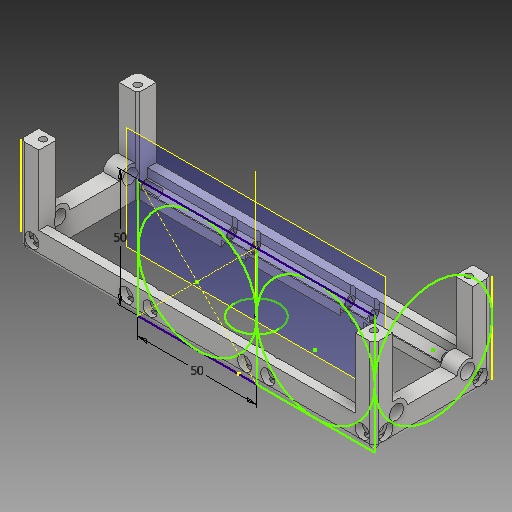
# Autodesk Inventor part: 10_Cube_2x_v0
Saved by Autodesk Inventor 2019 (Build 230136000, 136)
## iProperties
Created: 2018-05-19
Part Number: 10_Cube_2x_v0
Material: Generisch
Document SubType Name: Modeling
Designer: diederichbenedict
Density: 1 g/cm^3
Appearance: Vorgabe
Mass: 20.3218 g
Surface Area: 129.075 cm^2
Volume: 20.3218 cm^3
Author: diederichbenedict
Autodesk Inventor part; units mm, degrees
ref_plane "YZ Plane" through (0, 0, 0) normal (1, 0, 0) x (0, 1, 0)
ref_plane "XZ Plane" through (0, 0, 0) normal (0, 1, 0) x (-1, 0, 0)
sketch "Skizze1" plane through (0, 0, 0) normal (0, 0, 1) x (1, 0, 0)
  line L0 (-74.9, 24.9) -> (74.9, 24.9)
  line L1 (74.9, 24.9) -> (74.9, -24.9)
  line L2 (74.9, -24.9) -> (-74.9, -24.9)
  line L3 (-74.9, -24.9) -> (-74.9, 24.9)
  line L4 (-74.9, 24.9) -> (74.9, -24.9) construction
  line L5 (74.9, 24.9) -> (-74.9, -24.9) construction
  line L6 (66.9528, -17.9) -> (-66.9528, -17.9)
  line L7 (-67.9, -16.9528) -> (-67.9, 16.9528)
  line L8 (-66.9528, 17.9) -> (66.9528, 17.9)
  line L9 (67.9, 16.9528) -> (67.9, -16.9528)
  line L10 (20.5, -20.5) -> (-20.5, 20.5) construction
  line L11 (-20.5, -20.5) -> (20.5, 20.5) construction
  line L12 (-66.9528, 17.9) -> (-67.9, 16.9528)
  line L13 (-66.9528, 17.9) -> (-65.6133, 17.9) construction
  line L14 (67.9, -16.9528) -> (66.9528, -17.9)
  line L15 (67.9, -16.9528) -> (69.2395, -16.9528) construction
  line L16 (-67.9, -16.9528) -> (-66.9528, -17.9)
  line L17 (66.9528, 17.9) -> (67.9, 16.9528)
  point P0 (0, 0)
  dimension "d0" = 149.8
  dimension "d1" = 49.8
  dimension "d2" = 41
  dimension "d3" = 41
  dimension "d4" = 135
  dimension "d5" = 60
  dimension "d6" = 135
  dimension "d7" = 60
  dimension "a1" = 60
  dimension "d9" = 60
  dimension "a2" = 7
  dimension "d42" = 7
  dimension "d43" = 7
  dimension "d44" = 7
  constraints: 36 end point, 4 horizontal, 4 midpoint, 4 parallel, 4 perpendicular, 2 equal length
  measures "d0" distance of L1.end L2.end
  measures "d1" distance of L0.end L1.end
  measures "d2" distance of L10.end L11.end
  measures "d3" distance of L11.start L10.end
  measures "d4" angle of L12 L13
  measures "d5" distance from line of point (0, 0) L12
  measures "d6" angle of L14 L15
  measures "d7" distance from line of point (0, 0) L14
  measures "a1" distance from line of point (0, 0) L17
  measures "d9" distance from line of L16 point (0, 0)
  measures "a2" distance between parallel lines of L8 L0
  measures "d42" distance between parallel lines of L3 L7
  measures "d43" distance between parallel lines of L2 L6
  measures "d44" distance between parallel lines of L1 L9
extrude "Extrusion1" add sketch "Skizze1" along normal blind 10.3
sketch "Skizze2" plane through (0, 0, 10.3) normal (0, 0, 1) x (1, 0, 0)
  line L0 (-67.9, 16.9528) -> (-66.9528, 17.9) construction
  line L1 (-66.9528, 17.9) -> (66.9528, 17.9) construction
  line L2 (66.9528, 17.9) -> (67.9, 16.9528) construction
  line L3 (67.9, 16.9528) -> (67.9, -16.9528) construction
  line L4 (67.9, -16.9528) -> (66.9528, -17.9) construction
  line L5 (66.9528, -17.9) -> (-66.9528, -17.9) construction
  line L6 (-66.9528, -17.9) -> (-67.9, -16.9528) construction
  line L7 (-67.9, -16.9528) -> (-67.9, 16.9528) construction
  line L8 (74.9, 24.9) -> (-74.9, 24.9) construction
  line L9 (-74.9, 24.9) -> (-74.9, -24.9) construction
  line L10 (-74.9, -24.9) -> (74.9, -24.9) construction
  line L11 (74.9, -24.9) -> (74.9, 24.9) construction
  line L12 (-67.9, -16.9528) -> (-74.9, -16.9528)
  line L13 (-74.9, -24.9) -> (-74.9, 24.9) projected
  line L14 (-74.9, -16.9528) -> (-74.9, -24.9)
  line L15 (-67.9, -16.9528) -> (-66.9528, -17.9) projected
  line L16 (-67.9, -16.9528) -> (-66.9528, -17.9)
  line L17 (-66.9528, -17.9) -> (-66.9528, -24.9)
  line L18 (74.9, -24.9) -> (-74.9, -24.9) projected
  line L19 (-74.9, -24.9) -> (-66.9528, -24.9)
  line L20 (-17.9, -14.9) -> (-17.9, 14.9) projected
  line L21 (14.9, -17.9) -> (-14.9, -17.9) projected
  line L22 (17.9, 14.9) -> (17.9, -14.9) projected
  line L23 (-14.9, 17.9) -> (-9.9, 17.9) projected
  circle A0 centre (0, 0) radius 17.9
  line L24 (66.9528, -17.9) -> (67.9, -16.9528)
  line L25 (67.9, -16.9528) -> (74.9, -16.9528)
  line L26 (74.9, -24.9) -> (74.9, -16.9528)
  line L27 (66.9528, -24.9) -> (74.9, -24.9)
  line L28 (66.9528, -17.9) -> (66.9528, -24.9)
  line L29 (67.9, 16.9528) -> (66.9528, 17.9)
  line L30 (66.9528, 17.9) -> (66.9528, 24.9)
  line L31 (74.9, 24.9) -> (66.9528, 24.9)
  line L32 (74.9, 16.9528) -> (74.9, 24.9)
  line L33 (67.9, 16.9528) -> (74.9, 16.9528)
  line L34 (-66.9528, 17.9) -> (-67.9, 16.9528)
  line L35 (-67.9, 16.9528) -> (-74.9, 16.9528)
  line L36 (-74.9, 24.9) -> (-74.9, 16.9528)
  line L37 (-66.9528, 24.9) -> (-74.9, 24.9)
  line L38 (-66.9528, 17.9) -> (-66.9528, 24.9)
  line L39 (0, 0) -> (49.9, -49.9) construction
  line L40 (27.2236, -28.6378) -> (29.3449, -30.7591)
  line L41 (29.3449, -30.7591) -> (30.7591, -29.3449)
  line L42 (30.7591, -29.3449) -> (28.6378, -27.2236)
  line L43 (28.6378, -27.2236) -> (27.2236, -28.6378)
  line L44 (27.2236, -28.6378) -> (30.7591, -29.3449) construction
  line L45 (29.3449, -30.7591) -> (28.6378, -27.2236) construction
  line L46 (66.9528, -17.9) -> (67.9, -16.9528) projected
  point P0 (28.9914, -28.9914)
  point P1 (43.1335, -41.7193)
  point P2 (41.7193, -43.1335)
  dimension "d80" = 360
  dimension "d101" = 3
  dimension "d102" = 2
  constraints: 54 end point, 8 point on line, 3 perpendicular, 3 tangent, 2 collinear, 2 midpoint, 2 parallel, 1 centre point, 1 vertical, 3 other
  measures "d101" distance of L40.start L40.end
  measures "d102" distance of L41.end L40.end
extrude "Extrusion2" add sketch "Skizze2" along normal blind 29.4 contours L15 L17 L18 L13 L12 | L13 L37 L38 L34 L35 | L18 L28 L24 L25 L26 | L29 L30 L31 L32 L33
fillet "Rundung1" radius 2 8 edges at (74.9, 24.9, 19.85) (74.9, 0, 0) (74.9, -24.9, 19.85) (-74.9, 24.9, 19.85) (-74.9, -24.9, 19.85) (-74.9, 0, 0) (0, -24.9, 0) (0, 24.9, 0)
sketch "Skizze3" plane through (0, 0, 39.7) normal (0, 0, 1) x (1, 0, 0)
  line L0 (70, 20) -> (-70, 20) construction
  line L1 (-70, 20) -> (-70, -20) construction
  line L2 (-70, -20) -> (70, -20) construction
  line L3 (70, -20) -> (70, 20) construction
  line L4 (70, 20) -> (-70, -20) construction
  line L5 (-70, 20) -> (70, -20) construction
  line L6 (22.9, -22.9) -> (20.7681, -22.9) projected
  line L7 (22.9, -20.7681) -> (22.9, -22.9) projected
  arc A0 (20.7681, -22.9) -> (22.9, -20.7681) centre (20, -20) ccw projected
  point P0 (0, 0)
  point P1 (-20, 20)
  point P2 (-20, 20)
  point P3 (-20, 20)
  point P4 (20, -20)
  point P5 (20, -20)
  point P6 (-20, -20)
  point P7 (-20, 20)
  point P8 (20, -20)
  point P9 (-20, -20)
  point P10 (-20, 20)
  point P11 (-20, -20)
  point P12 (-20, 20)
  point P13 (-20, -20)
  point P14 (-20, 20)
  point P15 (-15.7881, 5.2)
  point P16 (-15.7881, -5.2)
  dimension "d15" = 140
  dimension "d16" = 40
  constraints: 12 end point, 2 midpoint, 2 parallel, 1 horizontal, 1 perpendicular
  measures "d15" distance of L2.end L1.end
  measures "d16" distance of L1.end L0.end
hole "Bohrung1" at (70, -20, 39.7) at (-70, -20, 39.7) at (-70, 20, 39.7) at (70, 20, 39.7) direction (0, 0, -1) diameter 2.9 depth 10 tip angle 118
sketch "Skizze4" plane through (0, 0, 0) normal (0, 0, -1) x (-1, 0, 0)
  line L0 (66.9528, 17.9) -> (67.9, 16.9528) projected
  line L1 (67.9, 16.9528) -> (67.9, -16.9528) projected
  line L2 (67.9, -16.9528) -> (66.9528, -17.9) projected
  line L3 (66.9528, -17.9) -> (-66.9528, -17.9) projected
  line L4 (-66.9528, -17.9) -> (-67.9, -16.9528) projected
  line L5 (-67.9, -16.9528) -> (-67.9, 16.9528) projected
  line L6 (-67.9, 16.9528) -> (-66.9528, 17.9) projected
  line L7 (-66.9528, 17.9) -> (66.9528, 17.9) projected
  line L8 (-72.9, 22.9) -> (72.9, 22.9) projected
  line L9 (-72.9, -22.9) -> (-72.9, 22.9) projected
  line L10 (72.9, -22.9) -> (-72.9, -22.9) projected
  line L11 (72.9, 22.9) -> (72.9, -22.9) projected
  line L12 (-70, 20) -> (70, 20) construction
  line L13 (70, 20) -> (70, -20) construction
  line L14 (70, -20) -> (-70, -20) construction
  line L15 (-70, -20) -> (-70, 20) construction
  line L16 (-70, 20) -> (70, -20) construction
  line L17 (70, 20) -> (-70, -20) construction
  line L18 (70, 20) -> (30, 20) construction
  line L19 (30, 20) -> (30, -20) construction
  line L20 (30, -20) -> (70, -20) construction
  line L21 (70, -20) -> (70, 20) construction
  line L22 (-70, 20) -> (-30, 20) construction
  line L23 (-30, 20) -> (-30, -20) construction
  line L24 (-30, -20) -> (-70, -20) construction
  line L25 (-70, -20) -> (-70, 20) construction
  line L26 (-30, -20) -> (30, -20) construction
  line L27 (30, -20) -> (30, 20) construction
  line L28 (30, 20) -> (-30, 20) construction
  line L29 (-30, 20) -> (-30, -20) construction
  line L30 (20, 20) -> (-20, 20) construction
  line L31 (-20, 20) -> (-20, -20) construction
  line L32 (-20, -20) -> (20, -20) construction
  line L33 (20, -20) -> (20, 20) construction
  line L34 (20, 20) -> (-20, -20) construction
  line L35 (-20, 20) -> (20, -20) construction
  point P0 (0, 0)
  dimension "d149" = 140
  dimension "d150" = 40
  dimension "d151" = 40
  dimension "d152" = 40
  dimension "d153" = 40
  dimension "d154" = 40
  constraints: 48 end point, 10 parallel, 5 horizontal, 5 perpendicular, 4 midpoint, 2 point on line
  measures "d149" distance of L13.end L14.end
  measures "d150" distance of L12.end L13.end
  measures "d151" distance of L20.end L19.end
  measures "d152" distance of L23.end L24.end
  measures "d153" distance of L32.end L31.end
  measures "d154" distance of L31.end L30.end
hole "Bohrung2" at (-70, 20, 0) at (-70, -20, 0) at (-30, -20, 0) at (-20, -20, 0) at (-30, 20, 0) at (-20, 20, 0) at (20, 20, 0) at (30, 20, 0) at (70, 20, 0) at (70, -20, 0) at (30, -20, 0) at (20, -20, 0) direction (0, 0, 1) diameter 3 depth 15 tip angle 118 counterbore diameter 6.2 counterbore depth 2.5
sketch "Skizze8" plane through (74.9, -16.9528, 10.3) normal (1, 0, 0) x (0, 0, -1)
  line L0 (8.3, 41.8528) -> (-29.4, 41.8528) projected
  line L1 (10.3, 38.0483) -> (10.3, 39.8528) projected
  line L2 (10.3, 39.8528) -> (8.3, 39.8528) projected
  line L3 (8.3, 39.8528) -> (8.3, -5.9472) projected
  line L4 (8.3, -5.9472) -> (10.3, -5.9472) projected
  line L5 (10.3, -5.9472) -> (10.3, -4.1426) projected
  line L6 (10.3, -1.9517) -> (10.3, 35.8574) projected
  line L7 (-29.4, -7.9472) -> (8.3, -7.9472) projected
  circle A0 centre (-14.6, 16.9528) radius 24.9 construction
  line L8 (-34.6, -3.0472) -> (5.4, -3.0472) construction
  line L9 (5.4, -3.0472) -> (5.4, 36.9528) construction
  line L10 (5.4, 36.9528) -> (-34.6, 36.9528) construction
  line L11 (-34.6, 36.9528) -> (-34.6, -3.0472) construction
  line L12 (-34.6, -3.0472) -> (5.4, 36.9528) construction
  line L13 (5.4, -3.0472) -> (-34.6, 36.9528) construction
  point P0 (-34.7, -4.2101)
  point P1 (5.3, 35.7899)
  point P2 (5.3, -4.2101)
  point P3 (-34.7, 35.7899)
  dimension "d155" = 40
  dimension "d156" = 40
  constraints: 12 end point, 3 tangent, 2 midpoint, 2 parallel, 2 vertical alignment, 1 centre point, 1 horizontal, 1 perpendicular
  measures "d155" distance of L10.end L9.end
  measures "d156" distance of L9.end L8.end
sketch "Skizze9" plane through (66.9528, 17.9, 10.3) normal (-1, 0, 0) x (0, 0, 1)
  line L0 (-3.2288, -37.966) -> (32.6288, -37.966) construction
  line L1 (32.6288, -37.966) -> (34.766, -35.8288) construction
  line L2 (34.766, -35.8288) -> (34.766, 0.0288) construction
  line L3 (34.766, 0.0288) -> (32.6288, 2.166) construction
  line L4 (32.6288, 2.166) -> (-3.2288, 2.166) construction
  line L5 (-3.2288, 2.166) -> (-5.366, 0.0288) construction
  line L6 (-5.366, 0.0288) -> (-5.366, -35.8288) construction
  line L7 (-5.366, -35.8288) -> (-3.2288, -37.966) construction
  circle A0 centre (29.7, -2.9) radius 3.2639 construction
  circle A1 centre (-0.3, -2.9) radius 3.2639 construction
  circle A2 centre (-0.3, -32.9) radius 3.2639 construction
  circle A3 centre (29.7, -32.9) radius 3.2639 construction
  circle A4 centre (14.7, -17.9) radius 13.3985 construction
  line L8 (-3.643, 3.166) -> (33.043, 3.166)
  line L9 (33.043, 3.166) -> (35.766, 0.443)
  line L10 (35.766, 0.443) -> (35.766, -36.243)
  line L11 (35.766, -36.243) -> (33.043, -38.966)
  line L12 (33.043, -38.966) -> (-3.643, -38.966)
  line L13 (-3.643, -38.966) -> (-6.366, -36.243)
  line L14 (-6.366, -36.243) -> (-6.366, 0.443)
  line L15 (-6.366, 0.443) -> (-3.643, 3.166)
  point P0 (-10.3, -17.9)
  dimension "d82" = 1
  constraints: 16 end point, 7 other
  measures "d82" distance between parallel lines of L4 L8
extrude "Extrusion5" cut sketch "Skizze9" along normal up to surface (133.9056 mm away)
sketch "Skizze10" plane through (-74.9, -16.9528, 10.3) normal (-1, 0, 0) x (0, 0, 1)
  circle A0 centre (-0.4, 31.4969) radius 3.0099 construction
  circle A1 centre (-0.4, 31.4969) radius 3.0099 projected
  circle A2 centre (-0.4, 1.497) radius 3.0099 projected
extrude "Extrusion6" cut sketch "Skizze10" against normal through all
sketch "Skizze11" plane through (-74.9, -22.9, 2) normal (-1, 0, 0) x (0, 0, 1)
  arc A0 (9.7049, 39.8528) -> (8.3, 34.4609) centre (7.9, 37.4441) ccw construction
  line L0 (9.7049, 39.8528) -> (37.7, 39.8528) construction
  line L1 (37.7, 45.8) -> (37.7, 39.8528) construction
  line L2 (0, 45.8) -> (37.7, 45.8) construction
  line L3 (0, 0) -> (0, 45.8) construction
  line L4 (37.7, 0) -> (0, 0) construction
  line L5 (37.7, 5.9472) -> (37.7, 0) construction
  line L6 (10.5113, 5.9472) -> (37.7, 5.9472) construction
  arc A1 (8.3, 10.4274) -> (10.5113, 5.9472) centre (7.9, 7.4442) ccw construction
  line L7 (8.3, 34.4609) -> (8.3, 10.4274) construction
  arc A2 (8.3, 34.4609) -> (9.7049, 39.8528) centre (7.9, 37.4441) ccw
  line L8 (10.5113, 5.9472) -> (37.7, 5.9472) projected
  line L9 (9.7049, 39.8528) -> (37.7, 39.8528) projected
  arc A3 (8.3, 33.1135) -> (11.5212, 39.8528) centre (7.9, 37.4441) ccw
  line L10 (8.3, 34.4609) -> (8.3, 10.4274) projected
  line L11 (8.3, 33.1135) -> (8.3, 34.4609)
  line L12 (11.5212, 39.8528) -> (9.7049, 39.8528)
  line L13 (8.3, 10.4274) -> (8.3, 34.4609) projected
  arc A4 (10.5113, 5.9472) -> (8.3, 10.4274) centre (7.9, 7.4442) ccw
  arc A5 (12.3275, 5.9472) -> (8.3, 12.1007) centre (7.9, 7.4442) ccw
  line L14 (8.3, 12.1007) -> (8.3, 10.4274)
  line L15 (12.3275, 5.9472) -> (10.5113, 5.9472)
  constraints: 9 point on circle, 8 end point, 4 centre point, 3 coincident, 2 collinear, 2 horizontal, 2 point on line
extrude "Extrusion7" add sketch "Skizze11" against normal up to surface (7 mm away)
sketch "Skizze12" plane through (74.9, -22.9, 2) normal (1, 0, 0) x (0, 0, -1)
  line L0 (-10.5113, 5.9472) -> (-37.7, 5.9472) projected
  arc A0 (-9.7049, 39.8528) -> (-6.0951, 39.8528) centre (-7.9, 37.4441) ccw projected
  line L1 (-9.7049, 39.8528) -> (-11.5212, 39.8528) projected
  arc A1 (-11.5212, 39.8528) -> (-8.3, 33.1135) centre (-7.9, 37.4441) ccw projected
  line L2 (-8.3, 12.1007) -> (-8.3, 33.1135) projected
  arc A2 (-8.3, 12.1007) -> (-12.3275, 5.9472) centre (-7.9, 7.4442) ccw projected
  line L3 (-10.5113, 5.9472) -> (-12.3275, 5.9472) projected
  arc A3 (-5.2888, 5.9472) -> (-10.5113, 5.9472) centre (-7.9, 7.4442) ccw projected
  line L4 (2, 5.9472) -> (-5.2888, 5.9472) projected
  line L5 (2, 39.8528) -> (2, 5.9472) projected
  line L6 (2, 39.8528) -> (-6.0951, 39.8528) projected
  line L7 (-8.3, 10.4274) -> (-8.3, 34.4609) projected
  point P0 (-8.3, -17.1828)
  constraints: 1 other
ref_plane "Arbeitsebene1" through (17.9, -21.066, 43) normal (-1, 0, 0) x (0, 0, 1)
extrude "Extrusion8" add sketch "Skizze12" against normal up to surface (7 mm away) contours L0 A2 L7 A3 | A1 L1 A0 L7
hole "Bohrung3" at (74.9, -21.163, 45) at (74.9, 18.837, 45) at (74.9, -20, 4.9) at (74.9, 20, 4.9) direction (-1, 0, 0) diameter 3 depth 15 tip angle 118 counterbore diameter 6.2 counterbore depth 2.5
sketch "Skizze14" plane through (0, 0, 0) normal (0, 0, -1) x (-1, 0, 0)
  circle A0 centre (0, 0) radius 9.428
  constraints: 1 centre point, 1 coincident
pattern_circular "Runde Anordnung3" count 2 over 360 about axis through (0, 0, 0) along (0, 0, 1) of "Bohrung3"
sketch "Skizze15" plane through (-66.9528, 24.9, 10.3) normal (0, 1, 0) x (1, 0, 0)
  line L0 (87.0528, -63.0868) -> (-2.9472, -63.0868) construction
  line L1 (-2.9472, -63.0868) -> (-2.9472, 5.25) construction
  line L2 (-2.9472, 5.25) -> (87.0528, 5.25) construction
  line L3 (87.0528, 5.25) -> (87.0528, -63.0868) construction
  line L4 (87.0528, -63.0868) -> (-2.9472, 5.25) construction
  line L5 (-2.9472, -63.0868) -> (87.0528, 5.25) construction
  circle A0 centre (-2.9472, 5.25) radius 2.5 construction
  circle A1 centre (87.0528, 5.25) radius 2.5 construction
  circle A2 centre (47.0528, 5.25) radius 2.5 construction
  circle A3 centre (37.0528, 5.25) radius 2.5 construction
  circle A4 centre (96.8528, 5.25) radius 2.9342
  circle A5 centre (136.8528, 5.25) radius 4.1581
  line L6 (141.8528, 8.3) -> (141.8528, 2.3) projected
  line L7 (-7.9472, 4.3046) -> (-7.9472, -29.4) projected
  point P0 (66.9528, 10.3)
  point P1 (42.0528, -28.9184)
  point P2 (141.8528, 4.3046)
  dimension "d134" = 90
  dimension "d135" = 5
  dimension "d136" = 5
  dimension "d137" = 5
  dimension "d138" = 5
  dimension "d139" = 40
  dimension "d140" = 40
  dimension "d157" = 5
  dimension "d158" = 40
  dimension "d159" = 5
  constraints: 12 end point, 6 centre point, 2 coincident, 2 midpoint, 2 parallel, 2 point on line, 1 horizontal, 1 perpendicular
  measures "d134" distance of L1.end L2.end
  measures "d135" diameter of A0
  measures "d136" diameter of A1
  measures "d137" diameter of A2
  measures "d138" diameter of A3
  measures "d139" distance from line of A3.centre L1
  measures "d140" distance from line of A2.centre L3
  measures "d157" distance from line of A5.centre L6
  measures "d158" distance of A4.centre A5.centre
  measures "d159" distance from line of L1.end L7
hole "Bohrung4" at (20.1, 24.9, 5.05) at (-19.9, 24.9, 5.05) at (-29.9, 24.9, 5.05) at (-69.9, 24.9, 5.05) at (29.9, 24.9, 5.05) at (69.9, 24.9, 5.05) direction (0, -1, 0) diameter 3 depth 8 tip angle 118 counterbore diameter 6 counterbore depth 3
ref_plane "Arbeitsebene2" through (0, 0, 0) normal (0, 1, 0) x (1, 0, 0)
mirror "Spiegeln1" about plane through (0, 0, 0) normal (0, 1, 0) of "Bohrung4"
sketch "Skizze16" plane through (74.9, 16.9528, 39.7) normal (1, 0, 0) x (0, 0, -1)
  line L0 (0, -41.8528) -> (37.7, -41.8528) projected
  line L1 (37.7, 7.9472) -> (0, 7.9472) projected
  circle A0 centre (14.8, -16.9528) radius 24.9
  constraints: 2 tangent, 1 centre point
sketch "Skizze17" plane through (-66.9528, -24.9, 10.3) normal (0, -1, 0) x (1, 0, 0)
  line L0 (-7.9472, 29.4) -> (-7.9472, -4.3046) projected
  line L1 (48.0483, -10.3) -> (85.8574, -10.3) projected
  line L2 (91.9528, 39.7) -> (41.9528, 39.7)
  line L3 (41.9528, 39.7) -> (41.9528, -10.3)
  line L4 (41.9528, -10.3) -> (91.9528, -10.3)
  line L5 (91.9528, -10.3) -> (91.9528, 39.7)
  line L6 (91.9528, 39.7) -> (41.9528, -10.3) construction
  line L7 (41.9528, 39.7) -> (91.9528, -10.3) construction
  circle A0 centre (66.9528, 14.7) radius 25
  line L8 (91.9528, 39.7) -> (141.9528, 39.7)
  line L9 (141.9528, 39.7) -> (141.9528, -10.3)
  line L10 (141.9528, -10.3) -> (91.9528, -10.3)
  line L11 (91.9528, -10.3) -> (91.9528, 39.7)
  circle A1 centre (116.9528, 14.7) radius 25
  point P0 (66.9528, 14.7)
  point P1 (84.6725, -10.3)
  dimension "d160" = 50
  dimension "d161" = 50
  constraints: 20 end point, 6 tangent, 4 parallel, 2 centre point, 2 horizontal, 2 midpoint, 2 perpendicular, 1 point on line
  measures "d160" distance of L4.end L3.end
  measures "d161" distance of L3.end L2.end
equation "\"d5\" = a1"
equation "\"d7\" = a1"
equation "\"d9\" = a1"
equation "\"d42\" = a2"
equation "\"d43\" = a2"
equation "\"d44\" = a2"
